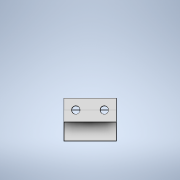
# Autodesk Inventor part: deadbolt enclosure wall holder bracket
Saved by Autodesk Inventor 2022 (Build 260153000, 153)
## iProperties
Created: 2022-04-10
Part Number: deadbolt enclosure wall holder bracket
Material: Generic
Document SubType Name: Modeling
Designer: a-dubs
Density: 1 g/cm^3
Appearance: Default
Author: a-dubs
Autodesk Inventor part; units mm, degrees
ref_plane "YZ Plane" through (0, 0, 0) normal (1, 0, 0) x (0, 1, 0)
ref_plane "XZ Plane" through (0, 0, 0) normal (0, 1, 0) x (-1, 0, 0)
ref_plane "XY Plane" through (0, 0, 0) normal (0, 0, 1) x (1, 0, 0)
sketch "Sketch1" plane through (0, 0, 0) normal (0, 1, 0) x (-1, 0, 0)
  line L0 (0, 0) -> (-9.6, 0)
  circle A0 centre (0, 0) radius 1.45
  circle A1 centre (-9.6, 0) radius 1.45
  line L1 (0, 0) -> (4, 0)
  line L2 (4, 0) -> (4, -4)
  line L3 (-9.6, 0) -> (-13.6, 0)
  line L4 (-13.6, 0) -> (-13.6, 4)
  line L5 (4, -4) -> (-13.6, -4)
  line L6 (-13.6, -4) -> (-13.6, 4)
  line L7 (-13.6, 4) -> (4, 4)
  line L8 (4, 4) -> (4, -4)
  line L9 (4, 4) -> (4, 10.4)
  line L10 (4, 10.4) -> (-13.6, 10.4)
  line L11 (-13.6, 10.4) -> (-13.6, 4)
  dimension "d0" = 9.6
  dimension "d1" = 2.9
  dimension "d4" = 4
  dimension "d7" = 6.4
  constraints: 24 end point, 4 perpendicular, 3 equal length, 3 horizontal, 2 centre point, 2 coincident, 2 parallel, 1 collinear, 1 equal radius, 1 point on line, 1 vertical
  measures "d0" distance of L0.start L0.end
  measures "d1" diameter of A0
  measures "d4" distance of L1.end L2.end
  measures "d7" distance of L7.end L9.end
extrude "Extrusion1" add sketch "Sketch1" along normal blind 6.4 contours A1 L3 L4 L7 L8 L1 A0 L0 | L0 A0 L1 L2 L5 L6 L3 A1
extrude "Extrusion2" add sketch "Sketch1" against normal blind 3.2 contours A1 L3 L4 L7 L8 L1 A0 L0 | L0 A0 L1 L2 L5 L6 L3 A1 | L11 L10 L9 L7
body "Solid1"
